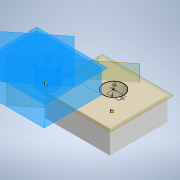
# Autodesk Inventor part: mascon
Saved by Autodesk Inventor 2021 (Build 250183000, 183)
## iProperties
Created: 2021-03-06
Part Number: mascon
Material: Generic
Document SubType Name: Modeling
Designer: ben
Density: 1 g/cm^3
Appearance: Default
Author: ben
Autodesk Inventor part; units mm, degrees
ref_plane "YZ Plane" through (0, 0, 0) normal (1, 0, 0) x (0, 1, 0)
ref_plane "XZ Plane" through (0, 0, 0) normal (0, 1, 0) x (-1, 0, 0)
ref_plane "XY Plane" through (0, 0, 0) normal (0, 0, 1) x (1, 0, 0)
sketch "Sketch1" plane through (0, 0, 0) normal (0, 1, 0) x (-1, 0, 0)
  line L0 (-90, -80) -> (90, -80)
  line L1 (90, -80) -> (90, 80)
  line L2 (90, 80) -> (-90, 80)
  line L3 (-90, 80) -> (-90, -80)
  line L4 (-90, -80) -> (90, 80) construction
  line L5 (90, -80) -> (-90, 80) construction
  point P0 (0, 0)
  dimension "d0" = 180
  dimension "d1" = 160
  constraints: 12 end point, 2 midpoint, 2 parallel, 1 horizontal, 1 perpendicular
  measures "d0" distance of L2.end L1.end
  measures "d1" distance of L1.end L0.end
extrude "Extrusion1" add sketch "Sketch1" along normal blind 100
sketch "Sketch2" plane through (0, 100, 0) normal (0, 1, 0) x (1, 0, 0)
  line L0 (-90, -80) -> (90, -80) projected
  line L1 (90, -80) -> (-20, -80)
  line L2 (-20, -80) -> (-20, 35)
  line L3 (-20, 35) -> (90, 35)
  line L4 (90, 35) -> (90, -80)
  line L5 (-90, 80) -> (-90, -80) projected
  line L6 (-90, -80) -> (-75, -80)
  line L7 (-75, -80) -> (-75, 80)
  line L8 (-75, 80) -> (-90, 80)
  line L9 (-90, 80) -> (-90, -80)
  point P0 (0, 0)
  dimension "d4" = 110
  dimension "d5" = 115
  dimension "d6" = 15
  dimension "d7" = 160
  constraints: 16 end point, 4 parallel, 2 horizontal, 2 perpendicular
  measures "d4" distance of L2.end L3.end
  measures "d5" distance of L1.end L2.end
  measures "d6" distance of L8.end L7.end
  measures "d7" distance of L7.end L6.end
extrude "Extrusion2" cut sketch "Sketch2" against normal blind 35
sketch "Sketch3" plane through (0, 65, 0) normal (0, 1, 0) x (1, 0, 0)
  circle A0 centre (0, 20) radius 28
  point P0 (0, 0)
  dimension "d10" = 56
  dimension "d11" = 0
  dimension "d12" = 20
  constraints: 1 centre point
  measures "d10" diameter of A0
  measures "d11" horizontal distance of A0.centre point (0, 0)
  measures "d12" distance of A0.centre point (0, 0)
extrude "Extrusion3" cut sketch "Sketch3" along normal blind 35 and the other way blind 35
ref_plane "Work Plane1" through (-45.0321, 105, -20) normal (-0.6217781, 0, -0.7831935) x (0, -1, 0)
sketch "Sketch5" plane through (-45.0321, 105, -20) normal (-0.6217781, 0, -0.7831935) x (0, -1, 0)
  line L0 (5, -13.8361) -> (5, 85.6484) projected
  arc A0 (5, 2.5) -> (2.5, 0) centre (5, 0) ccw
  line L1 (5, 0) -> (2.5, 0) construction
  line L2 (5, 0) -> (5, 2.5) construction
  line L3 (2.5, 0) -> (5, 0)
  line L4 (125.6036, 0) -> (-18.6213, 0) projected
  point P0 (105, -22.8333)
  dimension "d19" = 2.5
  dimension "d20" = 90
  constraints: 6 end point, 2 point on circle, 1 centre point, 1 collinear, 1 point on line
  measures "d19" radius of A0
  measures "d20" angle of L2 L1
revolve "Revolution1" add sketch "Sketch5" angle 360 about axis through (-45.0321, 105, -20) along (0, 1, 0)
pattern_circular "Circular Pattern1" count 4 over 90 about axis through (0, 65, -20) along (0, -1, 0) of "Revolution1"
body "Solid1"
